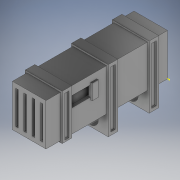
# Autodesk Inventor part: Part1
Saved by Autodesk Inventor 2021 (Build 250183000, 183)
## iProperties
Created: 2021-05-04
Part Number: Part1
Material: Generic
Document SubType Name: Modeling
Designer: AHUJA
Density: 1 g/cm^3
Appearance: Default
Author: AHUJA
Autodesk Inventor part; units mm, degrees
ref_plane "YZ Plane" through (0, 0, 0) normal (1, 0, 0) x (0, 1, 0)
ref_plane "XZ Plane" through (0, 0, 0) normal (0, 1, 0) x (-1, 0, 0)
ref_plane "XY Plane" through (0, 0, 0) normal (0, 0, 1) x (1, 0, 0)
sketch "Sketch1" plane through (0, 0, 0) normal (0, 0, 1) x (1, 0, 0)
  line L0 (0, 0) -> (50.8, 0)
  line L1 (50.8, 0) -> (50.8, 63.5)
  line L2 (50.8, 63.5) -> (0, 63.5)
  line L3 (0, 63.5) -> (0, 0)
  dimension "d0" = 63.5
  dimension "d1" = 50.8
  constraints: 8 end point, 2 parallel, 1 horizontal, 1 perpendicular
  measures "d0" distance of L0.end L1.end
  measures "d1" distance of L1.end L2.end
extrude "Extrusion1" add sketch "Sketch1" along normal blind 184.15
sketch "Sketch2" plane through (0, 0, 184.15) normal (0, 0, 1) x (1, 0, 0)
  line L0 (5.021, 56.896) -> (8.763, 56.896)
  line L1 (8.763, 56.896) -> (8.763, 6.604)
  line L2 (8.763, 6.604) -> (5.021, 6.604)
  line L3 (5.021, 6.604) -> (5.021, 56.896)
  line L4 (0, 63.5) -> (0, 0) projected
  line L5 (50.8, 63.5) -> (0, 63.5) projected
  line L6 (17.467, 56.896) -> (21.209, 56.896)
  line L7 (21.209, 56.896) -> (21.209, 6.604)
  line L8 (21.209, 6.604) -> (17.467, 6.604)
  line L9 (17.467, 6.604) -> (17.467, 56.896)
  line L10 (29.913, 56.896) -> (33.655, 56.896)
  line L11 (33.655, 56.896) -> (33.655, 6.604)
  line L12 (33.655, 6.604) -> (29.913, 6.604)
  line L13 (29.913, 6.604) -> (29.913, 56.896)
  line L14 (42.359, 56.896) -> (46.101, 56.896)
  line L15 (46.101, 56.896) -> (46.101, 6.604)
  line L16 (46.101, 6.604) -> (42.359, 6.604)
  line L17 (42.359, 6.604) -> (42.359, 56.896)
  line L18 (50.8, 0) -> (50.8, 63.5) projected
  dimension "d4" = 3.742
  dimension "d5" = 50.292
  dimension "d6" = 5.021
  dimension "d7" = 6.604
  dimension "d8" = 8.704
  dimension "d9" = 6.604
  dimension "d10" = 3.742
  dimension "d11" = 3.742
  dimension "d12" = 8.704
  dimension "d13" = 3.742
  dimension "d16" = 8.704
  constraints: 32 end point, 8 parallel, 4 horizontal, 4 perpendicular
  measures "d4" distance of L0.start L0.end
  measures "d5" distance of L0.end L1.end
  measures "d6" distance between parallel lines of L4 L3
  measures "d7" distance between parallel lines of L5 L0
  measures "d8" distance between parallel lines of L1 L9
  measures "d9" distance between parallel lines of L5 L6
  measures "d10" distance of L6.start L6.end
  measures "d11" distance of L10.start L10.end
  measures "d12" distance between parallel lines of L13 L7
  measures "d13" distance of L14.start L14.end
  measures "d16" distance between parallel lines of L17 L11
extrude "Extrusion2" cut sketch "Sketch2" against normal blind 100
sketch "Sketch3" plane through (0, 0, 0) normal (-1, 0, 0) x (0, 0, 1)
  line L0 (15.895, 66.04) -> (30.358, 66.04)
  line L1 (30.358, 66.04) -> (30.358, -28.667)
  line L2 (30.358, -28.667) -> (15.895, -28.667)
  line L3 (15.895, -28.667) -> (15.895, 66.04)
  line L4 (0, 63.5) -> (0, 0) projected
  line L5 (0, 63.5) -> (184.15, 63.5) projected
  line L6 (77.905, 66.04) -> (92.368, 66.04)
  line L7 (92.368, 66.04) -> (92.368, -28.667)
  line L8 (92.368, -28.667) -> (77.905, -28.667)
  line L9 (77.905, -28.667) -> (77.905, 66.04)
  line L10 (147.737, 66.04) -> (162.2, 66.04)
  line L11 (162.2, 66.04) -> (162.2, -2.54)
  line L12 (162.2, -2.54) -> (147.737, -2.54)
  line L13 (147.737, -2.54) -> (147.737, 66.04)
  dimension "d19" = 94.707
  dimension "d20" = 14.463
  dimension "d21" = 15.895
  dimension "d22" = 2.54
  dimension "d23" = 94.707
  dimension "d24" = 14.463
  dimension "d25" = 68.58
  dimension "d26" = 14.463
  dimension "d27" = 2.54
  dimension "d28" = 2.54
  dimension "d29" = 47.547
  dimension "d30" = 55.369
  constraints: 24 end point, 6 parallel, 3 horizontal, 3 perpendicular
  measures "d19" distance of L0.end L1.end
  measures "d20" distance of L0.start L0.end
  measures "d21" distance between parallel lines of L4 L3
  measures "d22" distance between parallel lines of L5 L0
  measures "d23" distance of L6.end L7.end
  measures "d24" distance of L6.start L6.end
  measures "d25" distance of L10.end L11.end
  measures "d26" distance of L10.start L10.end
  measures "d27" distance between parallel lines of L5 L10
  measures "d28" distance between parallel lines of L5 L6
  measures "d29" distance between parallel lines of L9 L1
  measures "d30" distance between parallel lines of L13 L7
ref_plane "Work Plane1" through (53.34, 0, 0) normal (1, 0, 0) x (0, 0, -1)
extrude "Extrusion3" add sketch "Sketch3" along normal blind 55.88 from surface at -53.34
sketch "Sketch4" plane through (-2.54, -28.667, 30.358) normal (-1, 0, 0) x (0, 0, 1)
  point P0 (-30.358, 28.667)
sketch "Sketch5" plane through (-2.54, -28.667, 30.358) normal (-1, 0, 0) x (0, 0, 1)
  line L0 (-10.738, 90.177) -> (-3.756, 90.177)
  line L1 (-3.756, 90.177) -> (-3.756, 4.938)
  line L2 (-3.756, 4.938) -> (-10.738, 4.938)
  line L3 (-10.738, 4.938) -> (-10.738, 90.177)
  line L4 (-14.463, 94.707) -> (-14.463, 0) projected
  line L5 (51.272, 90.177) -> (58.254, 90.177)
  line L6 (58.254, 90.177) -> (58.254, 4.938)
  line L7 (58.254, 4.938) -> (51.272, 4.938)
  line L8 (51.272, 4.938) -> (51.272, 90.177)
  line L9 (47.547, 94.707) -> (47.547, 0) projected
  line L10 (0, 94.707) -> (-14.463, 94.707) projected
  line L11 (62.01, 94.707) -> (47.547, 94.707) projected
  line L12 (121.666, 90.087) -> (127.547, 90.087)
  line L13 (127.547, 90.087) -> (127.547, 28.667)
  line L14 (127.547, 28.667) -> (121.666, 28.667)
  line L15 (121.666, 28.667) -> (121.666, 90.087)
  line L16 (117.379, 94.707) -> (117.379, 26.127) projected
  point P0 (-30.358, 28.667)
  dimension "d34" = 6.982
  dimension "d35" = 85.239
  dimension "d36" = 3.725
  dimension "d37" = 6.982
  dimension "d38" = 85.239
  dimension "d39" = 3.725
  dimension "d40" = 4.53
  dimension "d41" = 4.53
  dimension "d42" = 61.42
  dimension "d43" = 5.881
  dimension "d44" = 4.287
  constraints: 24 end point, 6 parallel, 3 horizontal, 3 perpendicular
  measures "d34" distance of L0.start L0.end
  measures "d35" distance of L0.end L1.end
  measures "d36" distance between parallel lines of L4 L3
  measures "d37" distance of L5.start L5.end
  measures "d38" distance of L5.end L6.end
  measures "d39" distance between parallel lines of L9 L8
  measures "d40" distance between parallel lines of L10 L0
  measures "d41" distance between parallel lines of L11 L5
  measures "d42" distance of L12.end L13.end
  measures "d43" distance of L12.start L12.end
  measures "d44" distance between parallel lines of L16 L15
extrude "Extrusion4" cut sketch "Sketch5" against normal blind 2.54
sketch "Sketch6" plane through (0, 0, 92.368) normal (-1, 0, 0) x (0, 0, 1)
  line L0 (14.937, 53.681) -> (24.354, 53.681)
  line L1 (24.354, 53.681) -> (24.354, 30.706)
  line L2 (24.354, 30.706) -> (14.937, 30.706)
  line L3 (14.937, 30.706) -> (14.937, 53.681)
  line L4 (0, -28.667) -> (0, 66.04) projected
  line L5 (0, 63.5) -> (55.369, 63.5) projected
  point P0 (-92.368, 0)
  dimension "d48" = 9.417
  dimension "d49" = 14.937
  dimension "d50" = 9.819
  dimension "d51" = 22.975
  constraints: 8 end point, 2 parallel, 1 horizontal, 1 perpendicular
  measures "d48" distance of L0.start L0.end
  measures "d49" distance between parallel lines of L4 L3
  measures "d50" distance between parallel lines of L5 L0
  measures "d51" distance of L2.end L0.start
extrude "Extrusion5" add sketch "Sketch6" along normal blind 1.905
sketch "Sketch7" plane through (0, 0, 92.368) normal (-1, 0, 0) x (0, 0, 1)
  line L0 (24.354, 30.706) -> (24.354, 53.681) projected
  line L1 (24.354, 50.479) -> (55.5483, 50.479)
  line L2 (55.5483, 50.479) -> (55.5483, 34.348)
  line L3 (55.5483, 34.348) -> (24.354, 34.348)
  line L4 (24.354, 34.348) -> (24.354, 50.479)
  line L5 (0, 63.5) -> (55.369, 63.5) projected
  point P0 (-92.368, 0)
  dimension "d54" = 13.021
  dimension "d55" = 16.131
  constraints: 8 end point, 2 parallel, 1 horizontal, 1 perpendicular, 1 point on line
  measures "d54" distance between parallel lines of L5 L1
  measures "d55" distance of L1.end L2.end
extrude "Extrusion6" cut sketch "Sketch7" against normal blind 6.926
sketch "Sketch8" plane through (-1.905, 53.681, 116.722) normal (0, 0, 1) x (1, 0, 0)
  point P0 (1.905, -53.681)
sketch "Sketch9" plane through (-1.905, 53.681, 116.722) normal (0, 0, 1) x (1, 0, 0)
  line L0 (1.905, -19.333) -> (6.926, -19.333) projected
  line L1 (6.926, -19.333) -> (5.021, -19.333)
  line L2 (5.021, -19.333) -> (5.021, -3.202)
  line L3 (5.021, -3.202) -> (6.926, -3.202)
  line L4 (6.926, -3.202) -> (6.926, -19.333)
  point P0 (1.905, -53.681)
  dimension "d58" = 16.131
  dimension "d59" = 1.905
  constraints: 8 end point, 2 parallel, 1 horizontal, 1 perpendicular
  measures "d58" distance of L1.end L2.end
  measures "d59" distance of L0.end L1.end
extrude "Extrusion7" cut sketch "Sketch9" against normal blind 9.417
sketch "Sketch10" plane through (53.34, 66.04, 15.895) normal (0, 0, -1) x (-1, 0, 0)
  circle A0 centre (28.738, -80.425) radius 12.0905
  line L0 (55.88, 0) -> (55.88, -94.707) projected
  line L1 (0, -94.707) -> (55.88, -94.707) projected
  point P0 (53.34, -66.04)
  dimension "d62" = 27.142
  dimension "d63" = 14.282
  dimension "d64" = 24.181
  constraints: 1 centre point
  measures "d62" distance from line of L0 A0.centre
  measures "d63" distance from line of L1 A0.centre
  measures "d64" diameter of A0
sketch "Sketch11" plane through (53.34, 66.04, 77.905) normal (0, 0, -1) x (-1, 0, 0)
  circle A0 centre (27.142, -80.425) radius 12.0905
  line L0 (0, -94.707) -> (55.88, -94.707) projected
  line L1 (0, 0) -> (0, -94.707) projected
  point P0 (53.34, -66.04)
  dimension "d65" = 24.181
  dimension "d66" = 14.282
  dimension "d67" = 27.142
  constraints: 1 centre point
  measures "d65" diameter of A0
  measures "d66" distance from line of L0 A0.centre
  measures "d67" distance from line of L1 A0.centre
extrude "Extrusion8" cut sketch "Sketch10" against normal blind 30
extrude "Extrusion9" cut sketch "Sketch11" against normal blind 30
sketch "Sketch12" plane through (0, 0, 0) normal (0, 0, -1) x (-1, 0, 0)
  line L0 (-25.449, 0) -> (-24.765, 0)
  line L1 (-24.765, 0) -> (-24.765, 0.127)
  line L2 (-24.765, 0.127) -> (-25.449, 0.127)
  line L3 (-25.449, 0.127) -> (-25.449, 0)
  line L4 (0, 63.5) -> (0, 0) projected
  dimension "d72" = 0.127
  dimension "d73" = 0.684
  dimension "d74" = 24.765
  constraints: 8 end point, 2 parallel, 1 horizontal, 1 perpendicular
  measures "d72" distance of L0.end L1.end
  measures "d73" distance of L1.end L2.end
  measures "d74" distance between parallel lines of L4 L1
extrude "Extrusion10" cut sketch "Sketch12" against normal blind 500
sketch "Sketch13" plane through (50.8, 0, 92.368) normal (1, 0, 0) x (0, 0, -1)
  point P0 (92.368, 0)
sketch "Sketch14" plane through (50.8, 0, 92.368) normal (1, 0, 0) x (0, 0, -1)
  line L0 (-55.369, 56.896) -> (-55.369, 6.604) projected
  line L1 (-24.354, 50.479) -> (-24.354, 34.348)
  line L2 (-55.369, 34.348) -> (-55.369, 50.479)
  line L3 (0, 63.5) -> (-55.369, 63.5) projected
  line L4 (-14.937, 53.681) -> (-24.354, 53.681)
  line L5 (-24.354, 53.681) -> (-24.354, 30.706)
  line L6 (-24.354, 30.706) -> (-14.937, 30.706)
  line L7 (-14.937, 30.706) -> (-14.937, 53.681)
  point P0 (92.368, 0)
  point P1 (-24.354, 50.479)
  point P2 (-24.354, 34.348)
  dimension "d77" = 31.015
  dimension "d80" = 9.819
  dimension "d81" = 9.417
  dimension "d82" = 22.975
  constraints: 12 end point, 3 parallel, 1 horizontal, 1 perpendicular, 1 point on line
  measures "d77" distance of L2.end L1.start
  measures "d80" distance between parallel lines of L3 L4
  measures "d81" distance of L4.start L4.end
  measures "d82" distance of L6.end L4.start
extrude "Extrusion11" add sketch "Sketch14" along normal mid plane 5.021
sketch "Sketch15" plane through (50.8, 0, 92.368) normal (1, 0, 0) x (0, 0, -1)
  line L0 (-55.369, 63.5) -> (-55.369, 0) projected
  line L1 (-24.354, 53.681) -> (-24.354, 30.706) projected
  line L2 (-55.369, 50.479) -> (-24.354, 50.479)
  line L3 (-24.354, 50.479) -> (-24.354, 34.348)
  line L4 (-24.354, 34.348) -> (-55.369, 34.348)
  line L5 (-55.369, 34.348) -> (-55.369, 50.479)
  line L6 (0, 63.5) -> (-55.369, 63.5) projected
  point P0 (92.368, 0)
  dimension "d85" = 16.131
  dimension "d86" = 13.021
  constraints: 8 end point, 2 parallel, 2 point on line, 1 horizontal, 1 perpendicular
  measures "d85" distance between parallel lines of L4 L2
  measures "d86" distance between parallel lines of L6 L2
extrude "Extrusion12" cut sketch "Sketch15" against normal blind 5.021
sketch "Sketch16" plane through (50.8, 30.706, 116.722) normal (0, 0, 1) x (1, 0, 0)
  line L0 (0, 3.642) -> (-4.699, 3.642) projected
  line L1 (-4.699, 3.642) -> (-2.794, 3.642)
  line L2 (-2.794, 3.642) -> (-2.794, 19.773)
  line L3 (-2.794, 19.773) -> (-4.699, 19.773)
  line L4 (-4.699, 19.773) -> (-4.699, 3.642)
  point P0 (-50.8, -30.706)
  point P1 (-2.794, 3.642)
  dimension "d89" = 16.131
  dimension "d90" = 1.905
  constraints: 8 end point, 2 parallel, 1 horizontal, 1 perpendicular
  measures "d89" distance of L1.end L2.end
  measures "d90" distance of L2.end L3.end
extrude "Extrusion13" cut sketch "Sketch16" against normal blind 9.417
sketch "Sketch17" plane through (50.8, 0, 92.368) normal (0, -1, 0) x (1, 0, 0)
  line L0 (-40.298, 34.057) -> (-10.502, 34.057)
  line L1 (-10.502, 34.057) -> (-10.502, 27.55)
  line L2 (-10.502, 27.55) -> (-40.298, 27.55)
  line L3 (-40.298, 27.55) -> (-40.298, 34.057)
  line L4 (0, 0) -> (0, 55.369) projected
  line L5 (-50.8, 0) -> (-50.8, 55.369) projected
  line L6 (2.54, 55.369) -> (-53.34, 55.369) projected
  line L7 (-40.298, -35.775) -> (-10.502, -35.775)
  line L8 (-10.502, -35.775) -> (-10.502, -42.282)
  line L9 (-10.502, -42.282) -> (-40.298, -42.282)
  line L10 (-40.298, -42.282) -> (-40.298, -35.775)
  line L11 (0, -62.01) -> (0, -14.463) projected
  line L12 (-50.8, -62.01) -> (-50.8, -14.463) projected
  line L13 (2.54, -14.463) -> (-53.34, -14.463) projected
  point P0 (-50.8, -92.368)
  dimension "d93" = 10.502
  dimension "d94" = 10.502
  dimension "d95" = 6.507
  dimension "d96" = 21.312
  dimension "d97" = 6.507
  dimension "d98" = 10.502
  dimension "d99" = 10.502
  dimension "d100" = 21.312
  constraints: 16 end point, 4 parallel, 2 horizontal, 2 perpendicular
  measures "d93" distance between parallel lines of L4 L1
  measures "d94" distance between parallel lines of L5 L3
  measures "d95" distance between parallel lines of L2 L0
  measures "d96" distance between parallel lines of L0 L6
  measures "d97" distance between parallel lines of L9 L7
  measures "d98" distance between parallel lines of L11 L8
  measures "d99" distance between parallel lines of L12 L10
  measures "d100" distance between parallel lines of L13 L7
extrude "Extrusion14" add sketch "Sketch17" along normal blind 2.54
sketch "Sketch18" plane through (53.34, -2.54, 147.737) normal (1, 0, 0) x (0, 0, -1)
  point P0 (147.737, 2.54)
sketch "Sketch19" plane through (53.34, -2.54, 147.737) normal (1, 0, 0) x (0, 0, -1)
  point P0 (147.737, 2.54)
sketch "Sketch20" plane through (53.34, -2.54, 147.737) normal (1, 0, 0) x (0, 0, -1)
  line L0 (-10.168, 63.96) -> (-4.287, 63.96)
  line L1 (-4.287, 63.96) -> (-4.287, 2.54)
  line L2 (-4.287, 2.54) -> (-10.168, 2.54)
  line L3 (-10.168, 2.54) -> (-10.168, 63.96)
  line L4 (-14.463, 68.58) -> (0, 68.58) projected
  line L5 (-14.463, 0) -> (-14.463, 68.58) projected
  line L6 (59.094, 63.642) -> (66.076, 63.642)
  line L7 (66.076, 63.642) -> (66.076, -21.597)
  line L8 (66.076, -21.597) -> (59.094, -21.597)
  line L9 (59.094, -21.597) -> (59.094, 63.642)
  line L10 (55.369, 68.58) -> (69.832, 68.58) projected
  line L11 (55.369, -26.127) -> (55.369, 68.58) projected
  line L12 (121.104, 63.642) -> (128.086, 63.642)
  line L13 (128.086, 63.642) -> (128.086, -21.597)
  line L14 (128.086, -21.597) -> (121.104, -21.597)
  line L15 (121.104, -21.597) -> (121.104, 63.642)
  line L16 (117.379, 68.58) -> (131.842, 68.58) projected
  line L17 (117.379, -26.127) -> (117.379, 68.58) projected
  point P0 (147.737, 2.54)
  dimension "d103" = 5.881
  dimension "d104" = 61.42
  dimension "d105" = 4.62
  dimension "d106" = 4.295
  dimension "d107" = 6.982
  dimension "d108" = 85.239
  dimension "d109" = 4.938
  dimension "d110" = 3.725
  dimension "d111" = 6.982
  dimension "d112" = 85.239
  dimension "d113" = 4.938
  dimension "d114" = 3.725
  constraints: 24 end point, 6 parallel, 3 horizontal, 3 perpendicular
  measures "d103" distance of L0.start L0.end
  measures "d104" distance of L0.end L1.end
  measures "d105" distance between parallel lines of L4 L0
  measures "d106" distance between parallel lines of L5 L3
  measures "d107" distance of L6.start L6.end
  measures "d108" distance of L6.end L7.end
  measures "d109" distance between parallel lines of L10 L6
  measures "d110" distance between parallel lines of L11 L9
  measures "d111" distance of L12.start L12.end
  measures "d112" distance of L12.end L14.start
  measures "d113" distance between parallel lines of L12 L16
  measures "d114" distance between parallel lines of L17 L15
extrude "Extrusion15" cut sketch "Sketch20" against normal blind 2.54
body "Solid1"
